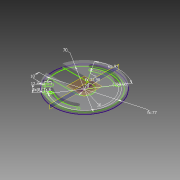
# Autodesk Inventor part: PorvedoRogzitesAVazhoz
Saved by Autodesk Inventor 2015 SP1 (Build 190203100, 203)
## iProperties
Created: 2014-11-14
Part Number: PorvedoRogzitesAVazhoz
Material: Polycarbonate, Clear
Document SubType Name: Modeling
Designer: laca
Density: 1.2 g/cm^3
Appearance: Polycarbonate - Clear
Mass: 15.8161 g
Surface Area: 87.1881 cm^2
Volume: 13.1801 cm^3
PorvedoRogzitesJatekSugara: 30.000 mm
Author: laca
Autodesk Inventor part; units mm, degrees
ref_plane "YZ Plane" through (0, 0, 0) normal (1, 0, 0) x (0, 1, 0)
ref_plane "XZ Plane" through (0, 0, 0) normal (0, 1, 0) x (-1, 0, 0)
ref_plane "XY Plane" through (0, 0, 0) normal (0, 0, 1) x (1, 0, 0)
sketch "Sketch1" plane through (0, 0, 0) normal (0, 1, 0) x (-1, 0, 0)
  circle A0 centre (0, 0) radius 38.5
  line L0 (0, 10) -> (0, -10)
  arc A1 (0, 10) -> (0, -10) centre (0, 0) ccw
  line L1 (0, -10) -> (37.1786, -10)
  line L2 (0, 10) -> (37.1786, 10)
  arc A2 (-16.3321, -25.1647) -> (16.3321, -25.1647) centre (0, 0) ccw construction
  arc A3 (-17.6931, -27.2618) -> (17.6931, -27.2618) centre (0, 0) ccw
  arc A4 (-14.9711, -23.0677) -> (14.9711, -23.0677) centre (0, 0) ccw
  arc A5 (-14.9711, -23.0677) -> (-17.6931, -27.2618) centre (-16.3321, -25.1647) ccw
  arc A6 (17.6931, -27.2618) -> (14.9711, -23.0677) centre (16.3321, -25.1647) ccw
  line L3 (16.3321, -25.1647) -> (0, 0)
  line L4 (0, 0) -> (-16.3321, -25.1647)
  arc A7 (17.6931, 27.2618) -> (-17.6931, 27.2618) centre (0, 0) ccw
  arc A8 (14.9711, 23.0677) -> (-14.9711, 23.0677) centre (0, 0) ccw
  arc A9 (14.9711, 23.0677) -> (17.6931, 27.2618) centre (16.3321, 25.1647) ccw
  arc A10 (-17.6931, 27.2618) -> (-14.9711, 23.0677) centre (-16.3321, 25.1647) ccw
  line L5 (29.3428, 20) -> (21.006, 28.6312)
  circle A11 centre (0, 0) radius 35
  line L6 (29.3428, 20) -> (25.0272, 15.8316) construction
  line L7 (27.9533, 21.4385) -> (23.6377, 17.2701)
  line L8 (26.4167, 14.3931) -> (30.7323, 18.5615)
  arc A12 (30.7323, 18.5615) -> (27.9533, 21.4385) centre (29.3428, 20) ccw
  arc A13 (23.6377, 17.2701) -> (26.4167, 14.3931) centre (25.0272, 15.8316) ccw
  line L9 (21.006, 28.6312) -> (16.6904, 24.4628) construction
  line L10 (19.6166, 30.0698) -> (15.3009, 25.9014)
  line L11 (18.0799, 23.0243) -> (22.3955, 27.1927)
  arc A14 (22.3955, 27.1927) -> (19.6166, 30.0698) centre (21.006, 28.6312) ccw
  arc A15 (15.3009, 25.9014) -> (18.0799, 23.0243) centre (16.6904, 24.4628) ccw
  point P0 (-10, 0)
  point P1 (25.1744, 24.3156)
  point P2 (27.185, 17.9158)
  point P3 (18.8482, 26.547)
  dimension "d49" = 70
  dimension "d7" = 20
  dimension "d10" = 77
  dimension "d13" = 5
  dimension "PorvedoRogzitesJatekSugara" = 30
  dimension "d25" = 65.968
  dimension "d26" = 32.984
  dimension "d29" = 360
  dimension "d45" = 12
  dimension "d52" = 6
  dimension "d53" = 10
  dimension "d54" = 2
  dimension "d55" = 2
  dimension "d56" = 6
  dimension "d57" = 6
  constraints: 31 point on circle, 28 end point, 15 centre point, 14 tangent, 4 midpoint, 3 coincident, 3 parallel, 3 perpendicular, 2 vertical, 27 other
  measures "d7" diameter of A1
  measures "d10" diameter of A0
  measures "d13" diameter of A6
  measures "PorvedoRogzitesJatekSugara" radius of A2
  measures "d25" angle of L4 L3
  measures "d26" angle of L0 L3
  measures "d45" distance of L5.start L5.end
  measures "d52" distance of L5.end point (25.174, 24.316)
  measures "d53" distance from line of L2 L5.start
  measures "d54" radius of A12
  measures "d55" radius of A14
  measures "d56" distance of L5.start L6.end
  measures "d57" distance of L5.end L9.end
ref_plane "Work Plane1" through (0, 0, 10) normal (-1, 0, 0) x (0, 0, -1)
ref_plane "Work Plane2" through (0, 3, 0) normal (0, 1, 0) x (1, 0, 0)
extrude "Extrusion5" add sketch "Sketch1" along normal blind 4 contours L2 A11 L8 A12 L5 A14 L10 L1 A0 | L2 A1 L4 A5 A3 A6 L3 L1 A11 L10 A7 A10 A8 A9 A15 L11 L7 A13 L8 | L8 A13 L7 A11 | A11 L7 A12 L8 | L3 A4 L4 A1 L1 | L10 A14 L11 A11 | A11 L11 A15 A9 A7 L10 | A11 L5 L7 | L11 L5 A11
extrude "Extrusion8" cut sketch "Sketch1" along normal blind 10 contours L8 A13 L7 A11 | A11 L7 A12 L8 | L10 A14 L11 A11 | A11 L11 A15 A9 A7 L10 | A7 A9 A15 L10
equation "\"d10\" = KulsoAtmeroPVCcso - 2 * PVCfalVastagsag"
equation "\"d26\" = 0.5 * d25"
equation "\"d55\" = d54"
equation "\"d57\" = d56"
equation "\"KulsoAtmeroPVCcso\" = 91"
equation "\"PVCfalVastagsag\" = 7"
body "Solid2"
